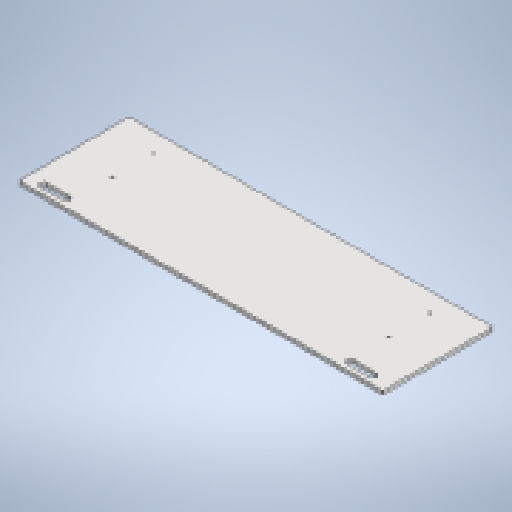
# Autodesk Inventor part: Plexi_Bildverarbeitungsband
Saved by Autodesk Inventor 2025 (Build 290162000, 162)
## iProperties
Created: 2025-08-17
Part Number: Plexi_Bildverarbeitungsband
Material: Generic
Document SubType Name: Modeling
Designer: peter
Density: 1 g/cm^3
Appearance: Default
Author: peter
Autodesk Inventor part; units mm, degrees
ref_plane "YZ Plane" through (0, 0, 0) normal (1, 0, 0) x (0, 1, 0)
ref_plane "XZ Plane" through (0, 0, 0) normal (0, 1, 0) x (-1, 0, 0)
ref_plane "XY Plane" through (0, 0, 0) normal (0, 0, 1) x (1, 0, 0)
sketch "Sketch1" plane through (0, 0, 0) normal (0, 0, 1) x (1, 0, 0)
  circle A0 centre (300, 45) radius 3 projected
  circle A1 centre (-300, -45) radius 3 projected
  circle A2 centre (300, -45) radius 3 projected
  circle A3 centre (-300, 45) radius 3 projected
  line L0 (395, -87) -> (-395, -87) projected
  line L1 (395, -87) -> (395, 87) projected
  line L2 (-395, 87) -> (395, 87) projected
  line L3 (-395, 87) -> (-395, -87) projected
  line L4 (395, 87) -> (-395, 87)
  line L5 (-395, 87) -> (-395, -148)
  line L6 (-395, -148) -> (395, -148)
  line L7 (395, -148) -> (395, 87)
  point P0 (0, 0)
  dimension "d0" = 235
  constraints: 8 end point, 2 parallel, 1 horizontal, 1 perpendicular, 1 vertical alignment
  measures "d0" distance of L5.end L4.end
extrude "Extrusion1" add sketch "Sketch1" along normal blind 8
sketch "Sketch2" plane through (0, 0, 8) normal (0, 0, 1) x (1, 0, 0)
  line L0 (387.8577, -133.54) -> (-386.877, -133.54) construction
  line L1 (390.6938, 247.5) -> (-382.1387, 247.5) construction
  arc A0 (355.5754, 239.7531) -> (355.5754, 255.2469) centre (355.5754, 247.5) ccw projected
  arc A1 (304.8389, 255.2469) -> (304.8389, 239.7531) centre (304.8389, 247.5) ccw projected
  line L2 (355.5754, 239.7531) -> (304.8389, 239.7531) projected
  line L3 (304.8389, 255.2469) -> (355.5754, 255.2469) projected
  line L4 (-310.6878, 239.7531) -> (-360.707, 239.7531) projected
  line L5 (-360.707, 255.2469) -> (-310.6878, 255.2469) projected
  arc A2 (-310.6878, 239.7531) -> (-310.6878, 255.2469) centre (-310.6878, 247.5) ccw projected
  arc A3 (-360.707, 255.2469) -> (-360.707, 239.7531) centre (-360.707, 247.5) ccw projected
  line L6 (304.8389, -133.54) -> (355.5754, -133.54) construction
  line L7 (304.8389, -141.2869) -> (355.5754, -141.2869)
  line L8 (355.5754, -125.7931) -> (304.8389, -125.7931)
  arc A4 (304.8389, -125.7931) -> (304.8389, -141.2869) centre (304.8389, -133.54) ccw
  arc A5 (355.5754, -141.2869) -> (355.5754, -125.7931) centre (355.5754, -133.54) ccw
  line L9 (-360.707, -133.54) -> (-310.6878, -133.54) construction
  line L10 (-360.707, -141.2869) -> (-310.6878, -141.2869)
  line L11 (-310.6878, -125.7931) -> (-360.707, -125.7931)
  arc A6 (-360.707, -125.7931) -> (-360.707, -141.2869) centre (-360.707, -133.54) ccw
  arc A7 (-310.6878, -141.2869) -> (-310.6878, -125.7931) centre (-310.6878, -133.54) ccw
  point P0 (0, 0)
  point P1 (330.2072, -133.54)
  point P2 (-335.6974, -133.54)
  dimension "d3" = 381.04
  constraints: 18 end point, 8 point on circle, 8 tangent, 4 centre point, 4 point on line, 2 midpoint, 2 parallel, 1 horizontal, 1 other
  measures "d3" distance between parallel lines of L0 L1
extrude "Extrusion2" cut sketch "Sketch2" against normal through all contours A4 L8 A5 L7 | A6 L11 A7 L10
thicken "Thicken1" operation add thickness 4 both sides no extend neighbours no toward (0, -1, 0) faces at (-131.6667, -148, 2.6667)
fillet "Fillet1" radius 2 4 edges at (395, -152, 4) (395, 87, 4) (-395, -152, 4) (-395, 87, 4)
body "Solid1"
